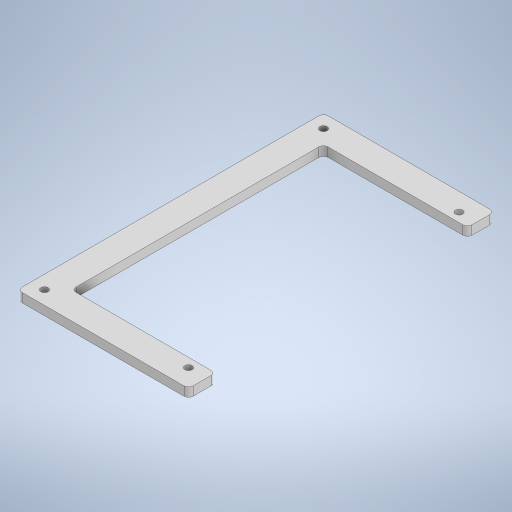
# Autodesk Inventor part: DB1-009
Saved by Autodesk Inventor 2023.4 (Build 274418000, 418)
## iProperties
Created: 2025-01-31
Part Number: DB1-009
Material: Generic
Document SubType Name: Modeling
Designer: 27karwoodwills
Density: 1 g/cm^3
Appearance: Default
Author: 27karwoodwills
Autodesk Inventor part; units mm, degrees
ref_plane "YZ Plane" through (0, 0, 0) normal (1, 0, 0) x (0, 1, 0)
ref_plane "XZ Plane" through (0, 0, 0) normal (0, 1, 0) x (-1, 0, 0)
ref_plane "XY Plane" through (0, 0, 0) normal (0, 0, 1) x (1, 0, 0)
sketch "Sketch1" plane through (0, 0, 0) normal (0, 1, 0) x (-1, 0, 0)
  line L0 (0, 0) -> (76.2, 0)
  line L1 (76.2, 0) -> (76.2, 19.05)
  line L2 (76.2, 19.05) -> (0, 19.05)
  line L3 (0, 19.05) -> (0, 0)
  line L4 (76.2, 19.05) -> (95.25, 19.05)
  line L5 (95.25, 19.05) -> (95.25, -196.85)
  line L6 (95.25, -196.85) -> (76.2, -196.85)
  line L7 (76.2, -196.85) -> (76.2, 19.05)
  line L8 (76.2, -196.85) -> (0, -196.85)
  line L9 (0, -196.85) -> (0, -177.8)
  line L10 (0, -177.8) -> (76.2, -177.8)
  line L11 (76.2, -177.8) -> (76.2, -196.85)
  line L12 (0, 0) -> (-25.4, 0)
  line L13 (-25.4, 0) -> (-25.4, 19.05)
  line L14 (-25.4, 19.05) -> (0, 19.05)
  line L15 (0, 19.05) -> (0, 0)
  line L16 (0, -177.8) -> (-25.4, -177.8)
  line L17 (-25.4, -177.8) -> (-25.4, -196.85)
  line L18 (-25.4, -196.85) -> (0, -196.85)
  line L19 (0, -196.85) -> (0, -177.8)
  circle A0 centre (-12.7, 6.35) radius 2.54
  circle A1 centre (-13.1033, -184.15) radius 2.54
  circle A2 centre (85.725, -187.325) radius 2.54
  circle A3 centre (85.725, 9.525) radius 2.54
  point P0 (76.2, -177.8)
  point P1 (-25.4, -187.325)
  point P2 (76.2, -187.325)
  dimension "d0" = 76.2
  dimension "d1" = 19.05
  dimension "d3" = 19.05
  dimension "d4" = 76.2
  dimension "d5" = 19.05
  dimension "d8" = 177.8
  dimension "d9" = 25.4
  dimension "d10" = 19.05
  dimension "d11" = 25.4
  dimension "d12" = 19.05
  dimension "d17" = 5.08
  dimension "d18" = 6.35
  dimension "d20" = 5.08
  dimension "d21" = 12.7
  dimension "d22" = 12.7
  dimension "d23" = 12.7
  dimension "d38" = 5.08
  dimension "d39" = 9.525
  dimension "d40" = 9.525
  dimension "d41" = 5.08
  dimension "d42" = 9.525
  dimension "d43" = 9.525
  constraints: 40 end point, 10 parallel, 5 horizontal, 5 perpendicular, 4 centre point, 4 coincident, 2 midpoint
  measures "d0" distance of L2.end L1.end
  measures "d1" distance of L1.end L0.end
  measures "d3" distance of L5.end L6.end
  measures "d4" distance of L9.end L10.end
  measures "d5" distance of L8.end L9.end
  measures "d8" distance between parallel lines of L10 L0
  measures "d9" distance of L13.end L14.end
  measures "d10" distance of L12.end L13.end
  measures "d11" distance of L18.end L17.end
  measures "d12" distance of L17.end L16.end
  measures "d17" diameter of A0
  measures "d18" distance from line of A0.centre L12
  measures "d20" diameter of A1
  measures "d21" distance from line of L18 A1.centre
  measures "d22" distance of point (-25.4, -187.325) A1.centre
  measures "d23" distance from line of point (-12.7, 6.35) L13
  measures "d38" diameter of A2
  measures "d39" distance from line of A2.centre L6
  measures "d40" distance of A2.centre point (76.2, -187.325)
  measures "d41" diameter of A3
  measures "d42" distance from line of L4 A3.centre
  measures "d43" distance from line of L5 A3.centre
extrude "Extrusion1" add sketch "Sketch1" along normal blind 6.35 contours L3 L2 L1 L0 | L12 L13 L14 L3 | L1 L4 L5 L6 L7 | L7 L8 L9 L10 | L9 L18 L17 L16 | A0 | A1 | A2 | A3
hole "Hole1" at (12.7, 0, 6.35) direction (0, 1, 0) diameter 5.1054 end through all clearance for "Flat Head Machine Screw (82)" size "#10" standard "Ansi Unified Screw Threads"
hole "Hole2" at (13.1033, 0, -184.15) direction (0, 1, 0) diameter 5.1054 end through all clearance for "Flat Head Machine Screw (82)" size "#10" standard "Ansi Unified Screw Threads"
hole "Hole3" at (-85.725, 0, -187.325) at (-85.725, 0, 9.525) direction (0, 1, 0) diameter 5.1054 end through all clearance for "Flat Head Machine Screw (82)" size "#10" standard "Ansi Unified Screw Threads"
fillet "Fillet1" radius 3.175 8 edges at (-95.25, 3.175, -196.85) (25.4, 3.175, -177.8) (25.4, 3.175, -196.85) (-76.2, 3.175, -177.8) (-76.2, 3.175, 0) (-95.25, 3.175, 19.05) (25.4, 3.175, 19.05) (25.4, 3.175, 0)
body "Solid1"
